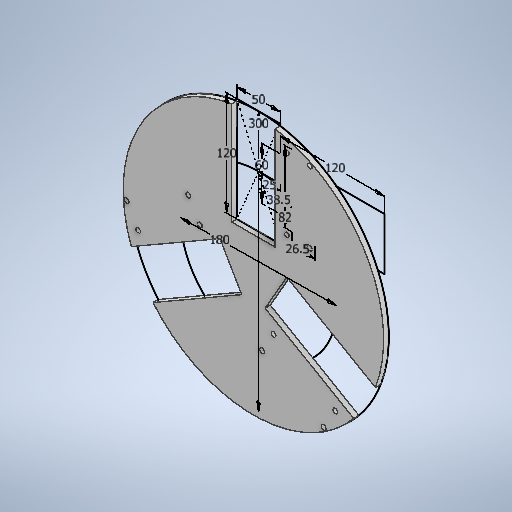
# Autodesk Inventor part: TempPart1
Saved by Autodesk Inventor 2025.3 (Build 293356000, 356)
## iProperties
Created: 2026-07-29
Part Number: TempPart1
Material: Generic
Document SubType Name: Modeling
Designer: louis
Density: 1 g/cm^3
Appearance: Default
Author: louis
Autodesk Inventor part; units mm, degrees
ref_plane "YZ Plane" through (0, 0, 0) normal (1, 0, 0) x (0, 1, 0)
ref_plane "XZ Plane" through (0, 0, 0) normal (0, 1, 0) x (-1, 0, 0)
ref_plane "XY Plane" through (0, 0, 0) normal (0, 0, 1) x (1, 0, 0)
sketch "Sketch1" plane through (0, 0, 0) normal (0, 1, 0) x (-1, 0, 0)
  circle A0 centre (0, 0) radius 90
  line L0 (-25, 120) -> (-25, 60)
  line L1 (-25, 60) -> (-145, 60)
  line L2 (-145, 60) -> (-145, 120)
  line L3 (-145, 120) -> (-25, 120)
  line L4 (-25, 90) -> (0, 90)
  line L5 (-65, 131) -> (-38.5, 131)
  line L6 (-38.5, 131) -> (-38.5, 49)
  line L7 (-38.5, 49) -> (-65, 49)
  line L8 (-65, 49) -> (-65, 131)
  line L9 (-38.5, 90) -> (-25, 90) construction
  circle A1 centre (0, 0) radius 150
  line L10 (-25, 30) -> (25, 30)
  line L11 (25, 30) -> (25, 150)
  line L12 (25, 150) -> (-25, 150)
  line L13 (-25, 150) -> (-25, 30)
  line L14 (-25, 30) -> (25, 150) construction
  line L15 (25, 30) -> (-25, 150) construction
  point P0 (-65, 62.2495)
  point P1 (-65, 60)
  point P2 (-67.082, 60)
  point P3 (25, 147.902)
  point P4 (-25, 147.902)
  dimension "d0" = 180
  dimension "d1" = 25
  dimension "d2" = 60
  dimension "d3" = 120
  dimension "d4" = 82
  dimension "d5" = 26.5
  dimension "d7" = 38.5
  dimension "d8" = 300
  dimension "d18" = 50
  dimension "d19" = 120
  constraints: 32 end point, 9 parallel, 6 coincident, 4 midpoint, 3 horizontal, 3 perpendicular, 1 centre point, 3 other
  measures "d1" distance of L4.start L4.end
  measures "d2" distance of L0.start L0.end
  measures "d3" distance of L2.end L0.start
  measures "d4" distance of L5.end L6.end
  measures "d5" distance of L6.end L7.end
  measures "d7" distance from line of L6 L4.end
  measures "d8" diameter of A1
  measures "d18" distance of L12.end L11.end
  measures "d19" distance of L11.end L10.end
extrude "Extrusion1" add sketch "Sketch1" against normal blind 6 contours A0 L1 L8 L7 L6 L13 L10 L11 | A0 L11 A1 L1 | L11 L10 L13 L0 A0 | A0 L4 L0 L13 A1 L11 | L1 A1 L3 L8 A0 | A0 L8 L1 | A0 L0 L4 | L8 L3 L6 A0 | A0 L6 L1 L8 | L1 L6 L7 L8 | L0 L1 L6 A0 | A0 L6 L3 L0 | L8 L5 L6 L3 | L3 A1 L13 L6 L5 L8
hole "Hole1" at (65, 0, 131) at (38.5, 0, 131) at (65, 0, 49) at (38.5, 0, 49) direction (0, -1, 0) diameter 5.6 end through all
extrude "Extrusion2" cut sketch "Sketch1" against normal blind 6 contours L11 L10 L13 L0 A0 | A0 L4 L0 L13 A1 L11 | A0 L0 L4
pattern_circular "Circular Pattern1" count 3 over 360 about axis through (0, 0, 0) along (0, -1, 0) of "Hole1", "Extrusion2"
body "Solid1"
